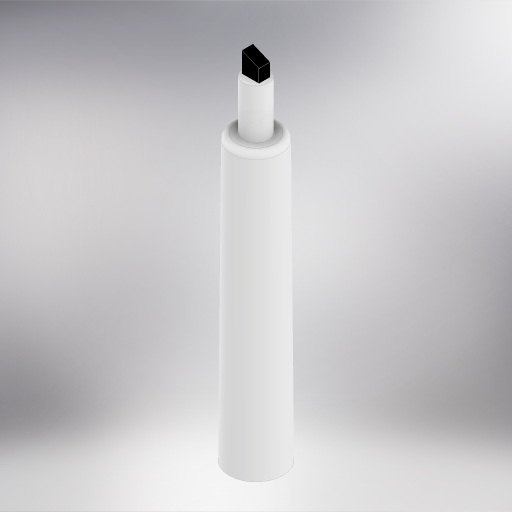
# Autodesk Inventor part: Marcador
Saved by Autodesk Inventor 2023 (Build 270158000, 158)
## iProperties
Created: 2023-02-27
Part Number: Marcador
Material: Madera (arce)
Document SubType Name: Modeling
Designer: Braya
Density: 0.67 g/cm^3
Appearance: Arce natural - De color oscuro brillante
Mass: 15.5555 g
Surface Area: 71.6173 cm^2
Volume: 23.2171 cm^3
Author: Braya
Autodesk Inventor part; units mm, degrees
ref_plane "YZ Plane" through (0, 0, 0) normal (1, 0, 0) x (0, 1, 0)
ref_plane "XY Plane" through (0, 0, 0) normal (0, 0, 1) x (1, 0, 0)
sketch "Boceto1" plane through (0, 0, 0) normal (0, 1, 0) x (-1, 0, 0)
  circle A0 centre (0, 0) radius 9.25
  dimension "d0" = 18.5
  constraints: 1 centre point, 1 coincident
  measures "d0" diameter of A0
ref_plane "Plano de trabajo1" through (0, 97.4, 0) normal (0, 1, 0) x (-1, 0, 0)
sketch "Boceto2" plane through (0, 97.4, 0) normal (0, 1, 0) x (-1, 0, 0)
  circle A0 centre (0, 0) radius 8.5
  dimension "d2" = 17
  constraints: 1 centre point, 1 coincident
  measures "d2" diameter of A0
loft "Solevación1" add profiles "Boceto2", "Boceto1"
sketch "Boceto3" plane through (0, 97.4, 0) normal (0, 1, 0) x (1, 0, 0)
  circle A0 centre (0, 0) radius 8.5 projected
  circle A1 centre (0, 0) radius 4.35
  dimension "d7" = 8.7
  constraints: 1 centre point, 1 coincident
  measures "d7" diameter of A1
extrude "Extrusión1" add sketch "Boceto3" along normal blind 17.1 contours A1
fillet "Empalme1" radius 2 1 edges at (8.5, 97.4, 0)
sketch "Boceto4" plane through (0, 114.5, 0) normal (0, 1, 0) x (1, 0, 0)
  line L0 (-2.95, -1.92) -> (2.95, -1.92)
  line L1 (2.95, -1.92) -> (2.95, 1.92)
  line L2 (2.95, 1.92) -> (-2.95, 1.92)
  line L3 (-2.95, 1.92) -> (-2.95, -1.92)
  line L4 (-2.95, -1.92) -> (2.95, 1.92) construction
  line L5 (2.95, -1.92) -> (-2.95, 1.92) construction
  point P0 (0, 0)
  dimension "d11" = 5.9
  dimension "d12" = 3.84
  constraints: 12 end point, 2 midpoint, 2 parallel, 1 horizontal, 1 perpendicular
  measures "d11" distance of L2.end L1.end
  measures "d12" distance of L1.end L0.end
extrude "Extrusión2" add sketch "Boceto4" along normal blind 4.5
sketch "Boceto5" plane through (-2.95, 114.5, 1.92) normal (0, 0, 1) x (1, 0, 0)
  line L0 (5.9, 4.5) -> (0, 4.5) projected
  line L1 (0, 4.5) -> (0, 7)
  line L2 (5.9, 0) -> (5.9, 4.5) projected
  line L3 (0, 7) -> (5.9, 4.5)
  line L4 (5.9, 4.5) -> (0, 4.5)
  point P0 (2.95, -114.5)
  dimension "d15" = 2.5
  constraints: 6 end point, 1 perpendicular, 1 vertical
  measures "d15" distance of L0.end L1.end
extrude "Extrusión3" add sketch "Boceto5" against normal up to surface (3.84 mm away)
sketch "Boceto6" plane through (0, 0, 0) normal (0, -1, 0) x (1, 0, 0)
  circle A0 centre (0, 0) radius 7
  line L0 (0, -7) -> (0, -4.3)
  line L1 (0, -4.3) -> (0.65, -4.3012)
  circle A1 centre (0, 0) radius 4.35 projected
  line L2 (0.65, -4.3012) -> (0.6452, -6.9702)
  line L3 (0, -4.3) -> (-0.65, -4.3)
  line L4 (0, -4.3) -> (0.65, -4.3) construction
  line L5 (-0.65, -4.3) -> (-0.65, -6.9698)
  line L6 (-2.5818, -3.501) -> (-4.4724, -5.3849)
  line L7 (-3.0406, -3.0406) -> (-2.5809, -3.5002) construction
  line L8 (-3.0406, -3.0406) -> (-3.5002, -2.5809)
  line L9 (-3.5002, -2.5809) -> (-5.388, -4.4687)
  line L10 (-3.0406, -3.0406) -> (-2.5818, -3.501)
  line L11 (-4.3012, -0.65) -> (-6.9702, -0.6452)
  line L12 (-4.3, 0) -> (-4.3, -0.65) construction
  line L13 (-4.3, 0) -> (-4.3, 0.65)
  line L14 (-4.3, 0.65) -> (-6.9698, 0.65)
  line L15 (-4.3, 0) -> (-4.3012, -0.65)
  line L16 (-3.501, 2.5818) -> (-5.3849, 4.4724)
  line L17 (-3.0406, 3.0406) -> (-3.5002, 2.5809) construction
  line L18 (-3.0406, 3.0406) -> (-2.5809, 3.5002)
  line L19 (-2.5809, 3.5002) -> (-4.4687, 5.388)
  line L20 (-3.0406, 3.0406) -> (-3.501, 2.5818)
  line L21 (-0.65, 4.3012) -> (-0.6452, 6.9702)
  line L22 (0, 4.3) -> (-0.65, 4.3) construction
  line L23 (0, 4.3) -> (0.65, 4.3)
  line L24 (0.65, 4.3) -> (0.65, 6.9698)
  line L25 (0, 4.3) -> (-0.65, 4.3012)
  line L26 (2.5818, 3.501) -> (4.4724, 5.3849)
  line L27 (3.0406, 3.0406) -> (2.5809, 3.5002) construction
  line L28 (3.0406, 3.0406) -> (3.5002, 2.5809)
  line L29 (3.5002, 2.5809) -> (5.388, 4.4687)
  line L30 (3.0406, 3.0406) -> (2.5818, 3.501)
  line L31 (4.3012, 0.65) -> (6.9702, 0.6452)
  line L32 (4.3, 0) -> (4.3, 0.65) construction
  line L33 (4.3, 0) -> (4.3, -0.65)
  line L34 (4.3, -0.65) -> (6.9698, -0.65)
  line L35 (4.3, 0) -> (4.3012, 0.65)
  line L36 (3.501, -2.5818) -> (5.3849, -4.4724)
  line L37 (3.0406, -3.0406) -> (3.5002, -2.5809) construction
  line L38 (3.0406, -3.0406) -> (2.5809, -3.5002)
  line L39 (2.5809, -3.5002) -> (4.4687, -5.388)
  line L40 (3.0406, -3.0406) -> (3.501, -2.5818)
  dimension "d18" = 14
  dimension "d19" = 2.7
  dimension "d20" = 0.65
  dimension "d21" = 90
  dimension "d22" = 0.65
  dimension "d23" = 180
  dimension "d24" = 90
  dimension "d27" = 360
  constraints: 82 end point, 3 coincident, 3 point on circle, 2 horizontal, 1 centre point, 1 collinear, 1 vertical, 97 other
  measures "d18" diameter of A0
  measures "d19" distance of L0.start L0.end
  measures "d20" distance of L0.end L1.end
  measures "d21" angle of L1 L2
  measures "d22" distance of L0.end L3.end
  measures "d23" angle of L3 L4
  measures "d24" angle of L5 L3
extrude "Extrusión4" cut sketch "Boceto6" against normal blind 10 contours L31 A1 L29 A0 | A0 L36 A1 L34 | L35 L33 A1 L40 L38 L1 L3 L10 L8 L15 L13 L20 L18 L25 L23 L30 L28 | L26 A1 L24 A0 | A0 L2 A1 L39 | L21 A1 L19 A0 | A0 L6 A1 L5 | L16 A1 L14 A0 | A0 L11 A1 L9
